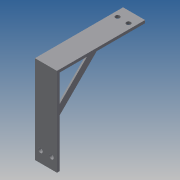
# Autodesk Inventor part: angleBracket
Saved by Autodesk Inventor 2014 SP1 (Build 180222100, 222)
## iProperties
Created: 2014-08-29
Part Number: angleBracket
Material: Generic
Document SubType Name: Modeling
Designer: Dave
Density: 1 g/cm^3
Appearance: Default
Author: Dave
Autodesk Inventor part; units mm, degrees
ref_plane "YZ Plane" through (0, 0, 0) normal (1, 0, 0) x (0, 1, 0)
ref_plane "XZ Plane" through (0, 0, 0) normal (0, 1, 0) x (-1, 0, 0)
sketch "Sketch1" plane through (0, 0, 0) normal (1, 0, 0) x (0, 1, 0)
  line L0 (0, 0) -> (101.6, 0)
  line L1 (101.6, 0) -> (101.6, -101.6)
  line L2 (98.425, -101.6) -> (98.425, -3.175)
  line L3 (98.425, -3.175) -> (0, -3.175)
  line L4 (101.6, -101.6) -> (98.425, -101.6)
  line L5 (0, 0) -> (0, -3.175)
  dimension "d0" = 101.6
  dimension "d1" = 101.6
  dimension "d2" = 3.175
  constraints: 12 end point, 3 perpendicular, 1 horizontal, 1 parallel, 1 other
  measures "d0" distance of L0.start L0.end
  measures "d1" distance of L0.end L1.end
  measures "d2" distance between parallel lines of L2 L1
extrude "Extrusion1" add sketch "Sketch1" along normal blind 25.4
ref_plane "Work Plane1" through (12.7, 0, 0) normal (1, 0, 0) x (0, 0, -1)
sketch "Sketch2" plane through (12.7, 0, 0) normal (1, 0, 0) x (0, 0, -1)
  line L0 (2.312, 31.3076) -> (70.5907, 99.5863)
  line L1 (2.312, 31.3076) -> (98.8727, 31.3076) construction
  line L2 (59.3736, 99.5863) -> (2.312, 42.5247)
  line L3 (70.5907, 99.5863) -> (59.3736, 99.5863)
  line L4 (2.312, 31.3076) -> (2.312, 42.5247)
  point P0 (0, 0)
  dimension "d6" = 45
  dimension "d7" = 7.9317
  constraints: 10 end point, 1 equal length, 1 horizontal, 1 perpendicular
  measures "d6" angle of L1 L0
  measures "d7" distance between parallel lines of L0 L2
extrude "Extrusion2" add sketch "Sketch2" along normal mid plane 1.778
sketch "Sketch4" plane through (0, 98.425, -101.6) normal (0, -1, 0) x (1, 0, 0)
  line L0 (0, 0) -> (0, 98.425) projected
  line L1 (0, 0) -> (25.4, 0) projected
  circle A0 centre (6.35, 12.7) radius 2.2746
  circle A1 centre (19.05, 12.7) radius 2.2746
  point P0 (0, 101.6)
  dimension "d10" = 12.7
  dimension "d11" = 6.35
  dimension "d14" = 12.7
  constraints: 2 centre point, 1 horizontal, 2 other
  measures "d10" distance from line of L1 A0.centre
  measures "d11" distance from line of L0 A0.centre
  measures "d14" distance of A0.centre A1.centre
hole "Hole1" at (19.05, 98.425, -88.9) at (6.35, 98.425, -88.9) direction (0, 1, 0) diameter 5.1054 depth 25.4 tip angle 118 clearance for "Flat Head Machine Screw (82)" size "#10" standard "Ansi Unified Screw Threads"
sketch "Sketch5" plane through (0, 0, -3.175) normal (0, 0, -1) x (-1, 0, 0)
  line L0 (-25.4, 0) -> (-25.4, 98.425) projected
  line L1 (0, 0) -> (-25.4, 0) projected
  circle A0 centre (-19.05, 12.7) radius 2.2861
  circle A1 centre (-6.35, 12.7) radius 2.2861
  dimension "d26" = 12.7
  dimension "d27" = 6.35
  dimension "d30" = 12.7
  constraints: 2 centre point, 1 horizontal, 2 other
  measures "d26" distance from line of L1 A0.centre
  measures "d27" distance from line of L0 A0.centre
  measures "d30" distance of A0.centre A1.centre
hole "Hole2" at (19.05, 12.7, -3.175) at (6.35, 12.7, -3.175) direction (0, 0, 1) diameter 5.1054 depth 25.4 tip angle 118 clearance for "Flat Head Machine Screw (82)" size "#10" standard "Ansi Unified Screw Threads"
equation "\"d11\" = 0.25 * d3"
equation "\"d14\" = 0.5 * d3"
equation "\"d27\" = 0.25 * d3"
equation "\"d30\" = 0.5 * d3"
equation "\"d5\" = -0.5 * d3"
equation "\"d3\" = 25.4"
body "Solid1"
